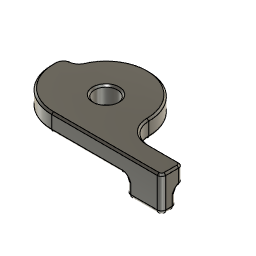
[a]_belt_tensioner_a_x2 (Autodesk Fusion 360 design; units mm, degrees)
Autodesk Fusion 360 part; units mm, degrees
sketch "Sketch1" plane through (0, 0, 0) normal (0, 0, 1) x (1, 0, 0) in component "[a]_belt_tensioner_a_x2"
  circle A0 centre (-3.5, 2.4) radius 2.7
  line L0 (19.5, -7.6) -> (19.5, -2.6)
  line L1 (19.5, -2.6) -> (11.5, -2.6)
  line L2 (19.5, -7.6) -> (-6.2, -7.6)
  arc A1 (6.5, 2.4) -> (11.5, -2.6) centre (11.5, 2.4) ccw
  line L3 (11.5, 2.4) -> (6.5, 2.4) construction
  line L4 (11.5, 2.4) -> (11.5, -2.6) construction
  arc A2 (6.5, 2.4) -> (-12.705, 6.3073) centre (-3.5, 2.4) ccw
  arc A3 (-14.3614, 5.0973) -> (-12.705, 6.3073) centre (-14.5461, 7.0888) ccw
  arc A4 (-14.3614, 5.0973) -> (-16.1723, 3.2378) centre (-14.1767, 3.1059) ccw
  arc A5 (-16.2, 2.4) -> (-6.2, -7.6) centre (-6.2, 2.4) ccw
  line L5 (-6.2, -7.6) -> (-6.2, 2.4) construction
  arc A6 (-16.1723, 3.2378) -> (-16.2, 2.4) centre (-3.5, 2.4) ccw
  line L6 (-16.2, 2.4) -> (-3.5, 2.4) construction
  point P0 (-3.5, 2.4)
  dimension "d1" = 5.4
  dimension "d2" = 90
  dimension "d3" = 2
  dimension "d4" = 2
  dimension "d5" = 10
  dimension "d6" = 10
  dimension "d7" = 5
  dimension "d8" = 10
  dimension "d10" = 23
  dimension "d12" = 3.5
  dimension "d14" = 2.4
  dimension "d15" = 12.7
  dimension "d16" = 157
  constraint coincident P0 A0.centre
  constraint vertical L0
  constraint perpendicular L0 L1
  constraint perpendicular L0 L2
  constraint tangent A2 A3
  constraint tangent L1 A1
  constraint tangent A1 A2
  constraint tangent A3 A4
  constraint coincident L2.end A5.end
  constraint tangent L2 A5
  constraint coincident A0 A5.centre
  constraint vertical L5
  constraint tangent A5 A6
  constraint tangent A0 L5
  constraint horizontal L6
  constraint tangent A4 A6
  measures "d1" diameter of A0
  measures "d2" angle of L3 L4
  measures "d3" radius of A3
  measures "d4" radius of A4
  measures "d5" distance of L2 P0
  measures "d6" radius of A2
  measures "d7" distance of L0.start L0.end
  measures "d8" radius of A5
  measures "d10" distance of P0 L0
  measures "d12" horizontal distance of origin A0.centre
  measures "d14" vertical distance of origin A0.centre
  measures "d15" radius of A6
  measures "d16" angle of P0 A1.start A2.end
extrude "Extrude1" add sketch "Sketch1" against normal blind 4 in component "[a]_belt_tensioner_a_x2"
sketch "Sketch2" plane through (0, 0, -4) normal (0, 0, -1) x (1, 0, 0) in component "[a]_belt_tensioner_a_x2"
  circle A0 centre (-3.5, -2.4) radius 2.7
  arc A1 (-16.1723, -3.2378) -> (-14.3614, -5.0973) centre (-14.1767, -3.1059) ccw
  arc A2 (-12.705, -6.3073) -> (-14.3614, -5.0973) centre (-14.5461, -7.0888) ccw
  arc A3 (-12.705, -6.3073) -> (6.5, -2.4) centre (-3.5, -2.4) ccw
  arc A4 (11.5, 2.6) -> (6.5, -2.4) centre (11.5, -2.4) ccw
  line L0 (11.5, 2.6) -> (19.5, 2.6)
  line L1 (19.5, 2.6) -> (19.5, 7.6)
  line L2 (19.5, 7.6) -> (-6.2, 7.6)
  arc A5 (-6.2, 7.6) -> (-16.2, -2.4) centre (-6.2, -2.4) ccw
  arc A6 (-16.2, -2.4) -> (-16.1723, -3.2378) centre (-3.5, -2.4) ccw
  line L3 (19.5, 7.6) -> (11.3, 7.6)
  line L4 (11.3, 7.6) -> (11.3, 4.1)
  line L5 (11.3, 4.1) -> (19.5, 4.1)
  line L6 (19.5, 4.1) -> (19.5, 7.6)
  dimension "d19" = 8.2
  dimension "d20" = 3.5
  constraint horizontal L3
  constraint vertical L4
  constraint horizontal L5
  constraint vertical L6
  constraint coincident L1.end L2.start
  measures "d19" distance of L1.end L3.end
  measures "d20" distance of L3.end L4.end
extrude "Extrude2" add sketch "Sketch2" along normal blind 4.4 contours L1 L2 L3 L4 L5 L6 in component "[a]_belt_tensioner_a_x2"
fillet "Fillet1" radius 1 11 edges at (19.5, -7.6, -4.2) (19.5, -2.6, -2) (19.5, -4.1, -6.2) (19.5, -5.85, -8.4) (15.4, -7.6, -8.4) (11.3, -5.85, -8.4) (15.4, -4.1, -8.4) (15.4, -4.1, -4) (11.3, -5.85, -4) (11.3, -4.1, -6.2) (11.3, -7.6, -6.2) in component "[a]_belt_tensioner_a_x2"
fillet "Fillet2" radius 0.6 12 edges at (11.5197, -7.6, -4.3197) (2.184, -7.6, -4) (-13.2711, -4.6711, -4) (-16.1931, 2.8191, -4) (-15.6095, 4.5012, -4) (-13.3663, 5.4738, -4) (-1.5063, 12.1992, -4) (7.9645, -1.1355, -4) (15, -2.6, -4) (19.1124, -2.8094, -4) (19.4921, -3.4747, -4.0046) (19.5, -4.417, -4.3882) in component "[a]_belt_tensioner_a_x2"
chamfer "Chamfer1" distance 0.4 angle 45 12 edges at (6.15, -7.6, 0) (-13.2711, -4.6711, 0) (-16.1931, 2.8191, 0) (-15.6095, 4.5012, 0) (-13.3663, 5.4738, 0) (-1.5063, 12.1992, 0) (7.9645, -1.1355, 0) (15, -2.6, 0) (19.2071, -2.8929, 0) (19.5, -5.1, 0) (19.2071, -7.3071, 0) (-6.0173, 3.3764, 0) in component "[a]_belt_tensioner_a_x2"
component "[a]_belt_tensioner_a_x2" placed x (1, 0, 0) y (0, 1, 0) z (0, 0, 1) at (0, 0, 0)
